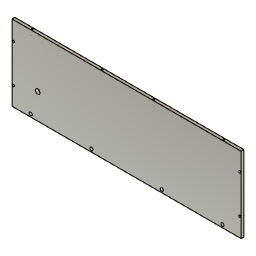
side_cover_front_wall v40 (Autodesk Fusion 360 design; units mm, degrees)
Autodesk Fusion 360 part; units mm, degrees
note: some values were not read from the file. Chosen so that the rebuilt part matches the saved one: which bodies a step acts on; which face or edge a step refers to; how an offset face is resized; which pieces of a blend or face edit are solid. Set by a fixed rule: which sketch regions a step uses.
sketch "Sketch1" plane through (0, 0, 0) normal (0, 1, 0) x (1, 0, 0)
  line L0 (0, 0) -> (470, 0)
  line L1 (470, 0) -> (470, -137.719)
  line L2 (470, -137.719) -> (0, -137.719)
  line L3 (0, -137.719) -> (0, 0)
  dimension "d1" = 470
  dimension "d2" = 137.719
  constraint horizontal L0
  constraint vertical L1
  constraint horizontal L2
  constraint vertical L3
  constraint coincident L0.start L3.end
  measures "d1" distance of L0.start L0.end
  measures "d2" distance of L0.start L2.end
extrude "Extrude1" add sketch "Sketch1" along normal blind 10 makes body 1
sketch "Sketch2" plane through (0, 0, 0) normal (0, -1, 0) x (1, 0, 0)
  line L0 (470, 137.719) -> (0, 137.719)
  line L1 (0, 137.719) -> (0, 0)
  line L2 (0, 0) -> (470, 0)
  line L3 (470, 0) -> (470, 137.719)
  line L4 (470, 0) -> (465, 0)
  line L5 (465, 0) -> (465, 25)
  line L6 (465, 25) -> (470, 25)
  line L7 (470, 25) -> (470, 0)
  line L8 (470, 137.719) -> (465, 137.719)
  line L9 (465, 137.719) -> (465, 112.719)
  line L10 (465, 112.719) -> (470, 112.719)
  line L11 (470, 112.719) -> (470, 137.719)
  line L12 (0, 137.719) -> (5, 137.719)
  line L13 (5, 137.719) -> (5, 112.719)
  line L14 (5, 112.719) -> (0, 112.719)
  line L15 (0, 112.719) -> (0, 137.719)
  line L16 (0, 0) -> (5, 0)
  line L17 (5, 0) -> (5, 25)
  line L18 (5, 25) -> (0, 25)
  line L19 (0, 25) -> (0, 0)
  dimension "d5" = 5
  dimension "d6" = 25
  dimension "d7" = 25
  dimension "d8" = 5
  dimension "d9" = 25
  dimension "d10" = 5
  dimension "d11" = 25
  constraint horizontal L4
  constraint vertical L5
  constraint horizontal L6
  constraint vertical L7
  constraint coincident L2.end L3.start
  constraint horizontal L8
  constraint vertical L9
  constraint horizontal L10
  constraint vertical L11
  constraint coincident L0.start L3.end
  constraint horizontal L12
  constraint vertical L13
  constraint horizontal L14
  constraint vertical L15
  constraint coincident L0.end L1.start
  constraint horizontal L16
  constraint vertical L17
  constraint horizontal L18
  constraint vertical L19
  constraint coincident L1.end L2.start
  measures "d5" distance of L2.end L4.end
  measures "d6" distance of L2.end L6.end
  measures "d7" distance of L0.start L10.end
  measures "d8" distance of L0.end L12.end
  measures "d9" distance of L0.end L14.end
  measures "d10" distance of L1.end L16.end
  measures "d11" distance of L1.end L18.end
sketch "Sketch3" plane through (0, 0, 137.719) normal (0, 0, 1) x (-1, 0, 0)
  line L0 (0, 0) -> (-470, 0)
  line L1 (-470, 0) -> (-470, -10)
  line L2 (-470, -10) -> (0, -10)
  line L3 (0, -10) -> (0, 0)
  line L4 (0, -5) -> (-60, -5)
  line L5 (-470, -5) -> (-410, -5)
  line L6 (-60, -5) -> (-235, -5)
  dimension "d15" = 60
  dimension "d16" = 60
  dimension "d17" = 175
  constraint midpoint L3 L4.start
  constraint perpendicular L3 L4
  constraint midpoint L1 L5.start
  constraint perpendicular L1 L5
  constraint parallel L5 L6
  measures "d15" distance of L4.start L4.end
  measures "d16" distance of L5.start L5.end
  measures "d17" distance of L4.end L6.end
extrude "Extrude2" cut 1 faces at (313.3333, 10, 91.8127) along direction (0, -1, 0) blind 4 on bodies 1 bodies 1
extrude "Extrude3" cut 1 faces at (470, 2, 45.9063) along direction (-1, 0, 0) blind 4 on bodies 1 bodies 1
extrude "Extrude4" cut 1 faces at (0, 2, 91.8127) along direction (1, 0, 0) blind 4 on bodies 1 bodies 1
sketch "Sketch4" plane through (4, 0, 0) normal (-1, 0, 0) x (0, -1, 0)
  line L0 (-6, 137.719) -> (-6, 0)
  line L1 (-6, 0) -> (0, 0)
  line L2 (0, 0) -> (0, 137.719)
  line L3 (0, 137.719) -> (-6, 137.719)
  line L4 (-3, 0) -> (-3, 25)
  line L5 (-3, 137.719) -> (-3, 112.719)
  dimension "d27" = 25
  dimension "d28" = 25
  constraint midpoint L1 L4.start
  constraint perpendicular L1 L4
  constraint midpoint L3 L5.start
  constraint perpendicular L3 L5
  measures "d27" distance of L4.start L4.end
  measures "d28" distance of L5.start L5.end
hole "Hole3" at (4, 3, 112.719) at (4, 3, 25) direction (1, 0, 0) diameter 3.332 depth 10 tip angle 180 bodies 1
thread "Thread3" "ISO Metric profile 4.0 M4x0.5 6H" major diameter 4.0861 minor diameter 3.5287 pitch 0.5 angle 60 resizes the face on face at (7.3333, 1.3345, 112.6775) on face at (7.3333, 3.083, 26.6639) on bodies 1
sketch "Sketch5" plane through (466, 0, 0) normal (1, 0, 0) x (0, 1, 0)
  line L0 (6, 0) -> (6, 137.719)
  line L1 (6, 137.719) -> (0, 137.719)
  line L2 (0, 137.719) -> (0, 0)
  line L3 (0, 0) -> (6, 0)
  line L4 (3, 0) -> (3, 25)
  line L5 (3, 137.719) -> (3, 112.719)
  dimension "d32" = 25
  dimension "d33" = 25
  constraint midpoint L3 L4.start
  constraint perpendicular L3 L4
  constraint midpoint L1 L5.start
  constraint perpendicular L1 L5
  measures "d32" distance of L4.start L4.end
  measures "d33" distance of L5.start L5.end
sketch "Sketch6" plane through (0, 0, 137.719) normal (0, 0, 1) x (-1, 0, 0)
  line L0 (-4, -6) -> (-4, 0)
  line L1 (-4, 0) -> (-466, 0)
  line L2 (-466, 0) -> (-466, -6)
  line L3 (-466, -6) -> (-4, -6)
  line L4 (-4, -3) -> (-64, -3)
  line L5 (-466, -3) -> (-406, -3)
  line L6 (-406, -3) -> (-235, -3)
  dimension "d37" = 60
  dimension "d38" = 60
  dimension "d39" = 171
  constraint midpoint L0 L4.start
  constraint perpendicular L0 L4
  constraint midpoint L2 L5.start
  constraint perpendicular L2 L5
  constraint parallel L3 L6
  measures "d37" distance of L4.start L4.end
  measures "d38" distance of L5.start L5.end
  measures "d39" distance of L5.end L6.end
delete_face "DeleteFace1" 1 faces at (10.6667, 1.2362, 112.763) on bodies 1
delete_face "DeleteFace2" 1 faces at (10.6667, 3.1757, 26.7556) on bodies 1
sketch "Sketch7" plane through (0, 6, 0) normal (0, 1, 0) x (-1, 0, 0)
  line L0 (-4, 0) -> (-4, 137.719)
  line L1 (-4, 137.719) -> (-466, 137.719)
  line L2 (-466, 137.719) -> (-466, 0)
  line L3 (-466, 0) -> (-4, 0)
  line L4 (-466, 137.719) -> (-463, 137.719)
  line L5 (-463, 137.719) -> (-463, 112.719)
  line L6 (-463, 112.719) -> (-466, 112.719)
  line L7 (-466, 112.719) -> (-466, 137.719)
  dimension "d43" = 3
  dimension "d44" = 25
  constraint horizontal L4
  constraint vertical L5
  constraint horizontal L6
  constraint vertical L7
  constraint coincident L1.end L2.start
  measures "d43" distance of L1.end L4.end
  measures "d44" distance of L1.end L6.end
hole "Hole6" at (463, 6, 112.719) direction (0, -1, 0) diameter 4.5 depth 80 tip angle 180 bodies 1
sketch "Sketch8" plane through (0, 6, 0) normal (0, 1, 0) x (-1, 0, 0)
  circle A0 centre (-463, 112.719) radius 2.25
  line L0 (-4, 0) -> (-4, 137.719)
  line L1 (-4, 137.719) -> (-466, 137.719)
  line L2 (-466, 137.719) -> (-466, 0)
  line L3 (-466, 0) -> (-4, 0)
  line L4 (-466, 0) -> (-463, 0)
  line L5 (-463, 0) -> (-463, 25)
  line L6 (-463, 25) -> (-466, 25)
  line L7 (-466, 25) -> (-466, 0)
  line L8 (-4, 137.719) -> (-7, 137.719)
  line L9 (-7, 137.719) -> (-7, 112.719)
  line L10 (-7, 112.719) -> (-4, 112.719)
  line L11 (-4, 112.719) -> (-4, 137.719)
  line L12 (-4, 0) -> (-7, 0)
  line L13 (-7, 0) -> (-7, 25)
  line L14 (-7, 25) -> (-4, 25)
  line L15 (-4, 25) -> (-4, 0)
  dimension "d48" = 3
  dimension "d49" = 25
  dimension "d50" = 3
  dimension "d51" = 25
  dimension "d52" = 3
  dimension "d53" = 25
  constraint horizontal L4
  constraint vertical L5
  constraint horizontal L6
  constraint vertical L7
  constraint coincident L2.end L3.start
  constraint horizontal L8
  constraint vertical L9
  constraint horizontal L10
  constraint vertical L11
  constraint coincident L0.end L1.start
  constraint horizontal L12
  constraint vertical L13
  constraint horizontal L14
  constraint vertical L15
  constraint coincident L0.start L3.end
  measures "d48" distance of L2.end L4.end
  measures "d49" distance of L2.end L6.end
  measures "d50" distance of L0.end L8.end
  measures "d51" distance of L0.end L10.end
  measures "d52" distance of L0.start L12.end
  measures "d53" distance of L0.start L14.end
extrude "Extrude5" cut 1 faces at (158, 2, 0) along direction (0, 0, 1) blind 4 on bodies 1 bodies 1
extrude "Extrude6" cut 1 faces at (158, 2, 4) along direction (0, 0, 1) blind 1 on bodies 1 bodies 1
sketch "Sketch9" plane through (0, 0, 5) normal (0, 0, -1) x (1, 0, 0)
  line L0 (4, 0) -> (4, -6)
  line L1 (4, -6) -> (466, -6)
  line L2 (466, -6) -> (466, 0)
  line L3 (466, 0) -> (4, 0)
  line L4 (466, -3) -> (406, -3)
  line L5 (406, -3) -> (235, -3)
  line L6 (235, -3) -> (64, -3)
  dimension "d61" = 60
  dimension "d62" = 171
  constraint midpoint L2 L4.start
  constraint perpendicular L2 L4
  constraint parallel L3 L5
  constraint perpendicular L0 L6
  measures "d61" distance of L4.start L4.end
  measures "d62" distance of L5.end L6.end
extrude "Extrude7" add 1 faces at (466, 2, 49.2397) along direction (1, 0, 0) blind 0.502 on bodies 1 bodies 1
delete_face "DeleteFace3" 1 faces at (462.4448, 4, 114.8994) on bodies 1
sketch "Sketch10" plane through (0, 0, 0) normal (0, -1, 0) x (1, 0, 0)
  line L0 (4, 5) -> (466.502, 5)
  line L1 (466.502, 5) -> (466.502, 137.719)
  line L2 (466.502, 137.719) -> (4, 137.719)
  line L3 (4, 137.719) -> (4, 5)
  line L4 (466.502, 137.719) -> (463.502, 137.719)
  line L5 (463.502, 137.719) -> (463.502, 112.719)
  line L6 (463.502, 112.719) -> (466.502, 112.719)
  line L7 (466.502, 112.719) -> (466.502, 137.719)
  line L8 (466.502, 5) -> (463.502, 5)
  line L9 (463.502, 5) -> (463.502, 30)
  line L10 (463.502, 30) -> (466.502, 30)
  line L11 (466.502, 30) -> (466.502, 5)
  dimension "d68" = 3
  dimension "d69" = 25
  dimension "d70" = 3
  dimension "d71" = 25
  constraint horizontal L4
  constraint vertical L5
  constraint horizontal L6
  constraint vertical L7
  constraint coincident L1.end L2.start
  constraint horizontal L8
  constraint vertical L9
  constraint horizontal L10
  constraint vertical L11
  constraint coincident L0.end L1.start
  measures "d68" distance of L1.end L4.end
  measures "d69" distance of L1.end L6.end
  measures "d70" distance of L0.end L8.end
  measures "d71" distance of L0.end L10.end
sketch "Sketch11" plane through (0, 0, 0) normal (0, -1, 0) x (1, 0, 0)
  line L0 (4, 5) -> (466.502, 5)
  line L1 (466.502, 5) -> (466.502, 137.719)
  line L2 (466.502, 137.719) -> (4, 137.719)
  line L3 (4, 137.719) -> (4, 5)
  line L4 (4, 5) -> (7, 5)
  line L5 (7, 5) -> (7, 30)
  line L6 (7, 30) -> (4, 30)
  line L7 (4, 30) -> (4, 5)
  dimension "d75" = 3
  dimension "d76" = 25
  constraint horizontal L4
  constraint vertical L5
  constraint horizontal L6
  constraint vertical L7
  constraint coincident L0.start L3.end
  measures "d75" distance of L0.start L4.end
  measures "d76" distance of L0.start L6.end
sketch "Sketch12" plane through (0, 0, 137.719) normal (0, 0, 1) x (-1, 0, 0)
  line L0 (-4, -6) -> (-4, 0)
  line L1 (-4, 0) -> (-466.502, 0)
  line L2 (-466.502, 0) -> (-466.502, -6)
  line L3 (-466.502, -6) -> (-4, -6)
  line L4 (-466.502, -3) -> (-406.502, -3)
  dimension "d80" = 60
  constraint midpoint L2 L4.start
  constraint perpendicular L2 L4
  measures "d80" distance of L4.start L4.end
sketch "Sketch13" plane through (0, 0, 137.719) normal (0, 0, 1) x (-1, 0, 0)
  line L0 (-4, -6) -> (-4, 0)
  line L1 (-4, 0) -> (-466.502, 0)
  line L2 (-466.502, 0) -> (-466.502, -6)
  line L3 (-466.502, -6) -> (-4, -6)
  line L4 (-64, -3) -> (-235.251, -3)
  dimension "d84" = 171.251
  constraint parallel L1 L4
  measures "d84" distance of L4.start L4.end
sketch "Sketch14" plane through (0, 0, 5) normal (0, 0, -1) x (1, 0, 0)
  line L0 (4, 0) -> (4, -6)
  line L1 (4, -6) -> (466.502, -6)
  line L2 (466.502, -6) -> (466.502, 0)
  line L3 (466.502, 0) -> (4, 0)
  line L4 (466.502, -3) -> (406.502, -3)
  dimension "d88" = 60
  constraint midpoint L2 L4.start
  constraint perpendicular L2 L4
  measures "d88" distance of L4.start L4.end
sketch "Sketch15" plane through (0, 0, 5) normal (0, 0, -1) x (1, 0, 0)
  line L0 (4, 0) -> (4, -6)
  line L1 (4, -6) -> (466.502, -6)
  line L2 (466.502, -6) -> (466.502, 0)
  line L3 (466.502, 0) -> (4, 0)
  line L4 (64, -3) -> (235.251, -3)
  dimension "d92" = 171.251
  constraint parallel L3 L4
  measures "d92" distance of L4.start L4.end
sketch "Sketch16" plane through (0, 0, 0) normal (0, -1, 0) x (1, 0, 0)
  line L0 (4, 5) -> (466.502, 5)
  line L1 (466.502, 5) -> (466.502, 137.719)
  line L2 (466.502, 137.719) -> (4, 137.719)
  line L3 (4, 137.719) -> (4, 5)
  line L4 (4, 5) -> (24, 5)
  line L5 (24, 5) -> (24, 11)
  line L6 (24, 11) -> (4, 11)
  line L7 (4, 11) -> (4, 5)
  line L8 (466.502, 5) -> (446.502, 5)
  line L9 (446.502, 5) -> (446.502, 11)
  line L10 (446.502, 11) -> (466.502, 11)
  line L11 (466.502, 11) -> (466.502, 5)
  line L12 (446.502, 11) -> (296.502, 11)
  line L13 (24, 11) -> (174, 11)
  dimension "d96" = 20
  dimension "d97" = 6
  dimension "d98" = 20
  dimension "d99" = 6
  dimension "d100" = 150
  dimension "d101" = 150
  constraint horizontal L4
  constraint vertical L5
  constraint horizontal L6
  constraint vertical L7
  constraint coincident L0.start L3.end
  constraint horizontal L8
  constraint vertical L9
  constraint horizontal L10
  constraint vertical L11
  constraint coincident L0.end L1.start
  constraint perpendicular L9 L12
  constraint perpendicular L5 L13
  measures "d96" distance of L0.start L4.end
  measures "d97" distance of L0.start L6.end
  measures "d98" distance of L0.end L8.end
  measures "d99" distance of L0.end L10.end
  measures "d100" distance of L9.end L12.end
  measures "d101" distance of L5.end L13.end
hole "Hole15" at (24, 0, 11) at (174, 0, 11) at (296.502, 0, 11) at (446.502, 0, 11) direction (0, 1, 0) diameter 6.6 depth 20 tip angle 180 bodies 1
extrude "Extrude8" add 1 faces at (312.3347, 2, 137.719) along direction (0, 0, 1) blind 13 on bodies 1 bodies 1
sketch "Sketch17" plane through (0, 0, 0) normal (0, -1, 0) x (1, 0, 0)
  circle A0 centre (296.502, 11) radius 3.3
  circle A1 centre (24, 11) radius 3.3
  circle A2 centre (174, 11) radius 3.3
  circle A3 centre (446.502, 11) radius 3.3
  line L0 (4, 5) -> (466.502, 5)
  line L1 (466.502, 5) -> (466.502, 150.719)
  line L2 (466.502, 150.719) -> (4, 150.719)
  line L3 (4, 150.719) -> (4, 5)
  line L4 (4, 5) -> (7, 5)
  line L5 (7, 5) -> (7, 25)
  line L6 (7, 25) -> (4, 25)
  line L7 (4, 25) -> (4, 5)
  line L8 (4, 150.719) -> (7, 150.719)
  line L9 (7, 150.719) -> (7, 130.719)
  line L10 (7, 130.719) -> (4, 130.719)
  line L11 (4, 130.719) -> (4, 150.719)
  line L12 (466.502, 150.719) -> (463.502, 150.719)
  line L13 (463.502, 150.719) -> (463.502, 130.719)
  line L14 (463.502, 130.719) -> (466.502, 130.719)
  line L15 (466.502, 130.719) -> (466.502, 150.719)
  line L16 (466.502, 5) -> (463.502, 5)
  line L17 (463.502, 5) -> (463.502, 25)
  line L18 (463.502, 25) -> (466.502, 25)
  line L19 (466.502, 25) -> (466.502, 5)
  dimension "d107" = 3
  dimension "d108" = 20
  dimension "d109" = 3
  dimension "d110" = 20
  dimension "d111" = 3
  dimension "d112" = 20
  dimension "d113" = 3
  dimension "d114" = 20
  constraint horizontal L4
  constraint vertical L5
  constraint horizontal L6
  constraint vertical L7
  constraint coincident L0.start L3.end
  constraint horizontal L8
  constraint vertical L9
  constraint horizontal L10
  constraint vertical L11
  constraint coincident L2.end L3.start
  constraint horizontal L12
  constraint vertical L13
  constraint horizontal L14
  constraint vertical L15
  constraint coincident L1.end L2.start
  constraint horizontal L16
  constraint vertical L17
  constraint horizontal L18
  constraint vertical L19
  constraint coincident L0.end L1.start
  measures "d107" distance of L0.start L4.end
  measures "d108" distance of L0.start L6.end
  measures "d109" distance of L2.end L8.end
  measures "d110" distance of L2.end L10.end
  measures "d111" distance of L1.end L12.end
  measures "d112" distance of L1.end L14.end
  measures "d113" distance of L0.end L16.end
  measures "d114" distance of L0.end L18.end
hole "Hole16" at (463.502, 0, 130.719) at (463.502, 0, 25) at (7, 0, 25) at (7, 0, 130.719) direction (0, 1, 0) diameter 4.5 depth 20 tip angle 180 bodies 1
delete_face "DeleteFace10" 1 faces at (172.4218, 2, 13.8981) on bodies 1
delete_face "DeleteFace11" 1 faces at (24.1645, 2, 7.7041) on bodies 1
delete_face "DeleteFace12" 1 faces at (7.224, 4, 22.7612) on bodies 1
delete_face "DeleteFace13" 1 faces at (4.7675, 2, 130.4392) on bodies 1
extrude "Extrude9" add 1 faces at (4, 2, 53.573) along direction (-1, 0, 0) blind 28 on bodies 1 bodies 1
sketch "Sketch18" plane through (0, 0, 0) normal (0, -1, 0) x (1, 0, 0)
  circle A0 centre (463.502, 130.719) radius 2.25
  circle A1 centre (463.502, 25) radius 2.25
  circle A2 centre (296.502, 11) radius 3.3
  circle A3 centre (446.502, 11) radius 3.3
  line L0 (-24, 5) -> (466.502, 5)
  line L1 (466.502, 5) -> (466.502, 150.719)
  line L2 (466.502, 150.719) -> (-24, 150.719)
  line L3 (-24, 150.719) -> (-24, 5)
  line L4 (-24, 5) -> (-21, 5)
  line L5 (-21, 5) -> (-21, 25)
  line L6 (-21, 25) -> (-24, 25)
  line L7 (-24, 25) -> (-24, 5)
  line L8 (-24, 150.719) -> (-21, 150.719)
  line L9 (-21, 150.719) -> (-21, 130.719)
  line L10 (-21, 130.719) -> (-24, 130.719)
  line L11 (-24, 130.719) -> (-24, 150.719)
  dimension "d120" = 3
  dimension "d121" = 20
  dimension "d122" = 3
  dimension "d123" = 20
  constraint horizontal L4
  constraint vertical L5
  constraint horizontal L6
  constraint vertical L7
  constraint coincident L0.start L3.end
  constraint horizontal L8
  constraint vertical L9
  constraint horizontal L10
  constraint vertical L11
  constraint coincident L2.end L3.start
  measures "d120" distance of L0.start L4.end
  measures "d121" distance of L0.start L6.end
  measures "d122" distance of L2.end L8.end
  measures "d123" distance of L2.end L10.end
hole "Hole17" at (-21, 0, 130.719) at (-21, 0, 25) direction (0, 1, 0) diameter 4.5 depth 20 tip angle 180 bodies 1
sketch "Sketch19" plane through (0, 0, 0) normal (0, -1, 0) x (1, 0, 0)
  circle A0 centre (-21, 130.719) radius 2.25
  circle A1 centre (-21, 25) radius 2.25
  circle A2 centre (463.502, 130.719) radius 2.25
  circle A3 centre (463.502, 25) radius 2.25
  circle A4 centre (296.502, 11) radius 3.3
  circle A5 centre (446.502, 11) radius 3.3
  line L0 (-24, 5) -> (466.502, 5)
  line L1 (466.502, 5) -> (466.502, 150.719)
  line L2 (466.502, 150.719) -> (-24, 150.719)
  line L3 (-24, 150.719) -> (-24, 5)
  line L4 (-24, 5) -> (-4, 5)
  line L5 (-4, 5) -> (-4, 11)
  line L6 (-4, 11) -> (-24, 11)
  line L7 (-24, 11) -> (-24, 5)
  line L8 (-4, 11) -> (146, 11)
  dimension "d127" = 20
  dimension "d128" = 6
  dimension "d129" = 150
  constraint horizontal L4
  constraint vertical L5
  constraint horizontal L6
  constraint vertical L7
  constraint coincident L0.start L3.end
  constraint perpendicular L5 L8
  measures "d127" distance of L0.start L4.end
  measures "d128" distance of L0.start L6.end
  measures "d129" distance of L5.end L8.end
hole "Hole18" at (-4, 0, 11) at (146, 0, 11) direction (0, 1, 0) diameter 6.6 depth 20 tip angle 180 bodies 1
extrude "Extrude10" add 1 faces at (139.5007, 4, 150.719) along direction (0, 0, 1) blind 12 on bodies 1 bodies 1
delete_face "DeleteFace14" 1 faces at (-23.2325, 2, 130.4392) on bodies 1
delete_face "DeleteFace15" 1 faces at (462.9468, 2, 128.5386) on bodies 1
sketch "Sketch20" plane through (0, 0, 0) normal (0, -1, 0) x (1, 0, 0)
  circle A0 centre (-4, 11) radius 3.3
  circle A1 centre (146, 11) radius 3.3
  circle A2 centre (-21, 25) radius 2.25
  circle A3 centre (463.502, 25) radius 2.25
  circle A4 centre (296.502, 11) radius 3.3
  circle A5 centre (446.502, 11) radius 3.3
  line L0 (-24, 5) -> (466.502, 5)
  line L1 (466.502, 5) -> (466.502, 162.719)
  line L2 (466.502, 162.719) -> (-24, 162.719)
  line L3 (-24, 162.719) -> (-24, 5)
  line L4 (466.502, 162.719) -> (463.502, 162.719)
  line L5 (463.502, 162.719) -> (463.502, 142.719)
  line L6 (463.502, 142.719) -> (466.502, 142.719)
  line L7 (466.502, 142.719) -> (466.502, 162.719)
  line L8 (-24, 162.719) -> (-21, 162.719)
  line L9 (-21, 162.719) -> (-21, 142.719)
  line L10 (-21, 142.719) -> (-24, 142.719)
  line L11 (-24, 142.719) -> (-24, 162.719)
  dimension "d135" = 3
  dimension "d136" = 20
  dimension "d137" = 3
  dimension "d138" = 20
  constraint horizontal L4
  constraint vertical L5
  constraint horizontal L6
  constraint vertical L7
  constraint coincident L1.end L2.start
  constraint horizontal L8
  constraint vertical L9
  constraint horizontal L10
  constraint vertical L11
  constraint coincident L2.end L3.start
  measures "d135" distance of L1.end L4.end
  measures "d136" distance of L1.end L6.end
  measures "d137" distance of L2.end L8.end
  measures "d138" distance of L2.end L10.end
hole "Hole19" at (-21, 0, 142.719) at (463.502, 0, 142.719) direction (0, 1, 0) diameter 4.5 depth 20 tip angle 180 bodies 1
sketch "Sketch21" plane through (0, 0, 162.719) normal (0, 0, 1) x (-1, 0, 0)
  line L0 (24, 0) -> (-466.502, 0)
  line L1 (-466.502, 0) -> (-466.502, -6)
  line L2 (-466.502, -6) -> (24, -6)
  line L3 (24, -6) -> (24, 0)
  line L4 (24, -3) -> (4, -3)
  line L5 (-466.502, -3) -> (-446.502, -3)
  line L6 (-446.502, -3) -> (-296.502, -3)
  line L7 (4, -3) -> (-146, -3)
  dimension "d142" = 20
  dimension "d143" = 20
  dimension "d144" = 150
  dimension "d145" = 150
  constraint midpoint L3 L4.start
  constraint perpendicular L3 L4
  constraint midpoint L1 L5.start
  constraint perpendicular L1 L5
  constraint parallel L5 L6
  constraint parallel L4 L7
  measures "d142" distance of L4.start L4.end
  measures "d143" distance of L5.start L5.end
  measures "d144" distance of L5.end L6.end
  measures "d145" distance of L4.end L7.end
sketch "Sketch22" plane through (0, 0, 0) normal (0, -1, 0) x (1, 0, 0)
  circle A0 centre (-21, 142.719) radius 2.25
  circle A1 centre (463.502, 142.719) radius 2.25
  circle A2 centre (-4, 11) radius 3.3
  circle A3 centre (146, 11) radius 3.3
  circle A4 centre (-21, 25) radius 2.25
  circle A5 centre (463.502, 25) radius 2.25
  circle A6 centre (296.502, 11) radius 3.3
  circle A7 centre (446.502, 11) radius 3.3
  line L0 (-24, 5) -> (466.502, 5)
  line L1 (466.502, 5) -> (466.502, 162.719)
  line L2 (466.502, 162.719) -> (-24, 162.719)
  line L3 (-24, 162.719) -> (-24, 5)
  line L4 (-4, 11) -> (16, 11)
  line L5 (446.502, 11) -> (426.502, 11)
  dimension "d149" = 20
  dimension "d150" = 20
  constraint coincident A2.centre L4.start
  constraint parallel L0 L4
  constraint coincident A7.centre L5.start
  constraint parallel L0 L5
  measures "d149" distance of A2.centre L4.end
  measures "d150" distance of A7.centre L5.end
hole "Hole21" at (426.502, 0, 11) at (16, 0, 11) direction (0, 1, 0) diameter 6.6 depth 10 tip angle 180 bodies 1
delete_face "DeleteFace16" 1 faces at (446.8306, 4, 7.7164) on bodies 1
delete_face "DeleteFace17" 1 faces at (-3.8355, 2, 7.7041) on bodies 1
sketch "Sketch23" plane through (0, 0, 0) normal (0, -1, 0) x (1, 0, 0)
  circle A0 centre (426.502, 11) radius 3.3
  circle A1 centre (16, 11) radius 3.3
  circle A2 centre (-21, 142.719) radius 2.25
  circle A3 centre (463.502, 142.719) radius 2.25
  circle A4 centre (146, 11) radius 3.3
  circle A5 centre (-21, 25) radius 2.25
  circle A6 centre (463.502, 25) radius 2.25
  circle A7 centre (296.502, 11) radius 3.3
  line L0 (-24, 5) -> (466.502, 5)
  line L1 (466.502, 5) -> (466.502, 162.719)
  line L2 (466.502, 162.719) -> (-24, 162.719)
  line L3 (-24, 162.719) -> (-24, 5)
  line L4 (-21, 25) -> (-21, 45)
  line L5 (-21, 142.719) -> (-21, 122.719)
  line L6 (463.502, 142.719) -> (463.502, 122.719)
  line L7 (463.502, 25) -> (463.502, 45)
  dimension "d154" = 20
  dimension "d155" = 20
  dimension "d156" = 20
  dimension "d157" = 20
  constraint coincident A5.centre L4.start
  constraint parallel L3 L4
  constraint coincident A2.centre L5.start
  constraint vertical L5
  constraint coincident A3.centre L6.start
  constraint perpendicular L2 L6
  constraint coincident A6.centre L7.start
  constraint parallel L1 L7
  measures "d154" distance of A5.centre L4.end
  measures "d155" distance of A2.centre L5.end
  measures "d156" distance of A3.centre L6.end
  measures "d157" distance of A6.centre L7.end
hole "Hole22" at (463.502, 0, 45) at (463.502, 0, 122.719) at (-21, 0, 45) at (-21, 0, 122.719) direction (0, 1, 0) diameter 4.5 depth 10 tip angle 180 bodies 1
delete_face "DeleteFace18" 1 faces at (-20.776, 4, 22.7612) on bodies 1
delete_face "DeleteFace19" 1 faces at (-23.2325, 2, 142.4392) on bodies 1
delete_face "DeleteFace20" 1 faces at (462.9468, 2, 140.5386) on bodies 1
delete_face "DeleteFace21" 1 faces at (462.9468, 2, 22.8196) on bodies 1
sketch "Sketch24" plane through (0, 0, 162.719) normal (0, 0, 1) x (-1, 0, 0)
  line L0 (24, 0) -> (-466.502, 0)
  line L1 (-466.502, 0) -> (-466.502, -6)
  line L2 (-466.502, -6) -> (24, -6)
  line L3 (24, -6) -> (24, 0)
  line L4 (-466.502, -3) -> (-426.502, -3)
  line L5 (-426.502, -3) -> (-276.502, -3)
  line L6 (24, -3) -> (-16, -3)
  line L7 (-16, -3) -> (-166, -3)
  dimension "d161" = 40
  dimension "d162" = 150
  dimension "d163" = 40
  dimension "d164" = 150
  constraint midpoint L1 L4.start
  constraint perpendicular L1 L4
  constraint parallel L4 L5
  constraint midpoint L3 L6.start
  constraint perpendicular L3 L6
  constraint parallel L6 L7
  measures "d161" distance of L4.start L4.end
  measures "d162" distance of L4.end L5.end
  measures "d163" distance of L6.start L6.end
  measures "d164" distance of L6.end L7.end
hole "Hole23" at (16, 3, 162.719) at (166, 3, 162.719) at (276.502, 3, 162.719) at (426.502, 3, 162.719) direction (0, 0, -1) diameter 3.332 depth 10 tip angle 180 bodies 1
thread "Thread12" "ISO Metric profile 4.0 M4x0.5 6H" major diameter 4.0861 minor diameter 3.5287 pitch 0.5 angle 60 resizes the face on face at (16.083, 1.3361, 159.3857) on face at (166.083, 1.3361, 159.3857) on face at (276.6679, 4.6577, 159.3857) on face at (426.6679, 4.6577, 159.3857) on bodies 1
ref_plane "WorkPlane1" through (221.251, 3, 82.719) normal (0, 0, 1) x (1, 0, 0)
split "Split1" by plane through (221.251, 3, 82.719) normal (0, 0, 1) bodies 1 makes body 2 at (141.2466, 0, 149.4641)
move_body "Move1" bodies 2 to x (1, 0, 0) y (0, 1, 0) z (0, 0, 1) at (0, 0, 4.281)
extrude "Extrude11" add 1 faces at (139.5007, 4, 82.719) along direction (0, 0, 1) blind 4.281 on bodies 1 bodies 1 2
sketch "Sketch25" plane through (0, 0, 0) normal (0, -1, 0) x (1, 0, 0)
  circle A0 centre (463.502, 127) radius 2.25
  circle A1 centre (-21, 127) radius 2.25
  line L0 (-24, 167) -> (-24, 5)
  line L1 (-24, 5) -> (466.502, 5)
  line L2 (466.502, 5) -> (466.502, 167)
  line L3 (466.502, 167) -> (-24, 167)
  circle A2 centre (-21, 45) radius 2.25
  circle A3 centre (463.502, 45) radius 2.25
  circle A4 centre (426.502, 11) radius 3.3
  circle A5 centre (16, 11) radius 3.3
  circle A6 centre (146, 11) radius 3.3
  circle A7 centre (296.502, 11) radius 3.3
  line L4 (-24, 5) -> (31, 5)
  line L5 (31, 5) -> (31, 60)
  line L6 (31, 60) -> (-24, 60)
  line L7 (-24, 60) -> (-24, 5)
  circle A8 centre (31, 60) radius 5
  dimension "d171" = 55
  dimension "d172" = 55
  dimension "d173" = 10
  constraint horizontal L4
  constraint vertical L5
  constraint horizontal L6
  constraint vertical L7
  constraint coincident L0.end L1.start
  constraint coincident L5.end L6.start
  measures "d171" distance of L0.end L4.end
  measures "d172" distance of L0.end L6.end
  measures "d173" diameter of A8
extrude "Extrude12" cut sketch "Sketch25" against normal blind 25 contours L5 L6 A8 | L5 L6 A8 bodies 1
equation "d17 = ( 350.000 / 2 ) * 1 mm"
equation "d39 = ( 342.000 / 2 ) * 1 mm"
equation "d62 = 231.000 mm - 60 mm"
equation "d84 = ( 342.502 / 2 ) * 1 mm"
equation "d92 = ( 342.502 / 2 ) * 1 mm"
